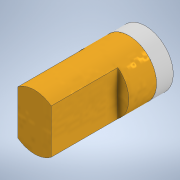
# Autodesk Inventor part: Вал
Saved by Autodesk Inventor 2022.3 (Build 263350000, 350)
## iProperties
Created: 2022-10-11
Part Number: Вал
Material: Типовые
Document SubType Name: Modeling
Designer: Admin
Density: 1 g/cm^3
Appearance: По умолчанию
Author: Admin
Autodesk Inventor part; units mm, degrees
ref_plane "YZ Plane" through (0, 0, 0) normal (1, 0, 0) x (0, 1, 0)
ref_plane "XZ Plane" through (0, 0, 0) normal (0, 1, 0) x (-1, 0, 0)
ref_plane "XY Plane" through (0, 0, 0) normal (0, 0, 1) x (1, 0, 0)
sketch "Эскиз1" plane through (0, 0, 0) normal (0, 0, 1) x (1, 0, 0)
  circle A0 centre (0, 0) radius 2.5
  line L0 (-1.5, 2) -> (-1.5, -2)
  line L1 (1.5, 2) -> (1.5, -2)
  line L2 (0, 0) -> (0, 0.8159) construction
  dimension "d0" = 5
  dimension "d1" = 3
  constraints: 6 end point, 4 point on circle, 2 vertical, 1 centre point, 1 coincident, 1 parallel, 1 other
  measures "d0" diameter of A0
  measures "d1" distance between parallel lines of L0 L1
extrude "Выдавливание1" add sketch "Эскиз1" against normal blind 2.5
extrude "Выдавливание2" add sketch "Эскиз1" along normal blind 6 contours L1 A0 L0
sketch "Эскиз2" plane through (0, 0, -2.5) normal (0, 0, -1) x (-1, 0, 0)
  circle A0 centre (0, 0) radius 2.5 projected
extrude "Выдавливание3" add sketch "Эскиз2" along normal blind 1.5 separate body
